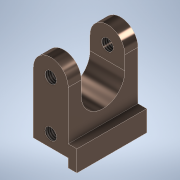
# Autodesk Inventor part: 7. 砲座
Saved by Autodesk Inventor 2022 (Build 260153000, 153)
## iProperties
Created: 2023-05-19
Part Number: 7. 砲座
Material: 一般
Document SubType Name: Modeling
Designer: USER
Density: 1 g/cm^3
Appearance: 砲銅 - 古董色拋光
Author: USER
Autodesk Inventor part; units mm, degrees
ref_plane "YZ Plane" through (0, 0, 0) normal (1, 0, 0) x (0, 1, 0)
ref_plane "XZ Plane" through (0, 0, 0) normal (0, 1, 0) x (-1, 0, 0)
ref_plane "XY Plane" through (0, 0, 0) normal (0, 0, 1) x (1, 0, 0)
sketch "草圖1" plane through (0, 0, 0) normal (1, 0, 0) x (0, 1, 0)
  arc A0 (0, 12.5) -> (0, -12.5) centre (0, 0) ccw
  line L0 (-27, 0) -> (-27, -20)
  line L1 (-27, -20) -> (18, -20)
  line L2 (18, 20) -> (-27, 20)
  line L3 (-27, 20) -> (-27, 0)
  line L4 (0, 12.5) -> (18, 12.5)
  line L5 (18, -12.5) -> (0, -12.5)
  line L6 (18, -12.5) -> (18, -20)
  line L7 (18, 12.5) -> (18, 20)
  dimension "d5" = 25
  dimension "d12" = 18
  dimension "d13" = 45
  dimension "d15" = 40
  dimension "d16" = 45
  dimension "d17" = 7.5
  dimension "d18" = 7.5
  dimension "d19" = 18
  constraints: 16 end point, 2 perpendicular, 2 point on circle, 2 tangent, 1 centre point, 1 coincident, 1 horizontal, 1 point on line, 1 vertical
  measures "d5" diameter of A0
  measures "d12" distance of L4.start L4.end
  measures "d13" distance of L0.end L1.end
  measures "d15" distance of L0.end L2.end
  measures "d16" distance of L2.end L2.start
  measures "d17" distance of L4.end L2.start
  measures "d18" distance of L5.start L1.end
  measures "d19" distance of L5.end L5.start
extrude "擠出1" add sketch "草圖1" along normal mid plane 20
sketch "草圖2" plane through (-10, -27, 20) normal (0, 0, 1) x (1, 0, 0)
  line L0 (20, 0) -> (20, 45) projected
  line L1 (20, 0) -> (20, 7)
  line L2 (20, 7) -> (25, 7)
  line L3 (25, 7) -> (25, 0)
  line L4 (25, 0) -> (25, -5)
  line L5 (25, -5) -> (20, -5)
  line L6 (0, 0) -> (20, 0) projected
  line L7 (20, -5) -> (20, 0)
  point P0 (10, 27)
  dimension "d22" = 7
  dimension "d23" = 5
  dimension "d24" = 5
  constraints: 12 end point, 4 perpendicular, 2 point on line
  measures "d22" distance of L0.start L1.end
  measures "d23" distance of L1.end L2.end
  measures "d24" distance of L3.end L4.end
extrude "擠出2" add sketch "草圖2" against normal up to surface (40 mm away)
fillet "圓角1" radius 10 4 edges at (10, 18, 16.25) (-10, 18, 16.25) (10, 18, -16.25) (-10, 18, -16.25)
sketch "草圖3" plane through (10, -32, 20) normal (0, 0, 1) x (1, 0, 0)
  line L0 (-20, 5) -> (0, 5) projected
  point P0 (-10, 32)
  point P1 (-10, 40)
  dimension "d30" = 35
  measures "d30" distance from line of L0 point (-10, 40)
hole "孔1" at (0, 8, 20) direction (0, 0, -1) diameter 6.647 end through all thread size "M8x1.25" class "6H" standard "ISO Metric profile"
sketch "草圖4" plane through (10, -32, 20) normal (0, 0, 1) x (1, 0, 0)
  line L0 (-20, 5) -> (0, 5) projected
  point P0 (-10, 32)
  point P1 (-10, 12)
  dimension "d38" = 7
  measures "d38" distance from line of L0 point (-10, 12)
hole "孔2" at (0, -20, 20) direction (0, 0, -1) diameter 6.647 depth 12 tip angle 118 thread size "M8x1.25" class "6H" standard "ISO Metric profile"
mirror "鏡射1" about plane through (0, 0, 0) normal (0, 0, 1) of "孔2"
sketch "草圖5" plane through (-10, -27, -20) normal (0, -1, 0) x (1, 0, 0)
  point P0 (10, 20)
  point P1 (10, 20)
  constraints: 1 coincident
hole "孔3" at (0, -27, 0) direction (0, 1, 0) diameter 4.917 depth 12 tip angle 118 thread size "M6x1" class "6H" standard "ISO Metric profile"
